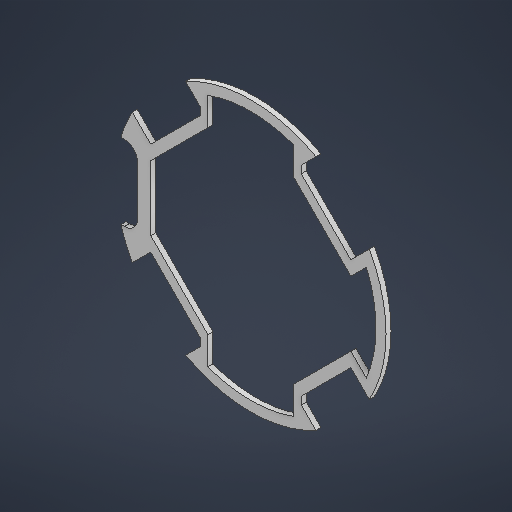
# Autodesk Inventor part: Part1
Saved by Autodesk Inventor 2026.1 (Build 301233020, 233B)
## iProperties
Created: 2026-04-01
Part Number: Part1
Material: Generic
Document SubType Name: Modeling
Designer: Bahaa
Density: 1 g/cm^3
Appearance: Default
Author: Bahaa
Autodesk Inventor part; units mm, degrees
ref_plane "YZ Plane" through (0, 0, 0) normal (1, 0, 0) x (0, 1, 0)
ref_plane "XZ Plane" through (0, 0, 0) normal (0, 1, 0) x (-1, 0, 0)
ref_plane "XY Plane" through (0, 0, 0) normal (0, 0, 1) x (1, 0, 0)
sketch "Sketch1" plane through (0, 0, 0) normal (0, 1, 0) x (-1, 0, 0)
  circle A0 centre (0, 0) radius 107.5
  line L0 (132.5, 30) -> (82.5, 30)
  line L1 (82.5, 30) -> (82.5, -30)
  line L2 (82.5, -30) -> (132.5, -30)
  line L3 (132.5, -30) -> (132.5, 30)
  line L4 (132.5, 30) -> (82.5, -30) construction
  line L5 (82.5, 30) -> (132.5, -30) construction
  line L6 (107.5, 30) -> (107.5, -30) construction
  line L7 (140.5, 38) -> (74.5, 38)
  line L8 (74.5, 38) -> (74.5, -38)
  line L9 (74.5, -38) -> (140.5, -38)
  line L10 (140.5, -38) -> (140.5, 38)
  line L11 (82.5, 0) -> (74.5, 0) construction
  line L12 (78.5, 0) -> (78.5, -18) construction
  line L13 (78.5, 0) -> (78.5, 18) construction
  line L14 (55.5079, 55.5079) -> (68.2358, 42.78) construction
  line L15 (55.5079, 55.5079) -> (42.78, 68.2358) construction
  line L16 (58.3363, 58.3363) -> (52.6795, 52.6795) construction
  line L17 (37.1231, 79.5495) -> (79.5495, 37.1231)
  line L18 (25.8094, 79.5495) -> (79.5495, 25.8094)
  line L19 (54.8008, 97.2272) -> (97.2272, 54.8008) construction
  line L20 (72.4784, 114.9049) -> (37.1231, 79.5495)
  line L21 (79.5495, 37.1231) -> (114.9049, 72.4784)
  line L22 (79.5495, 25.8094) -> (126.2186, 72.4784)
  line L23 (72.4784, 126.2186) -> (25.8094, 79.5495)
  line L24 (72.4784, 114.9049) -> (79.5495, 37.1231) construction
  line L25 (37.1231, 79.5495) -> (114.9049, 72.4784) construction
  line L26 (114.9049, 72.4784) -> (72.4784, 114.9049)
  line L27 (126.2186, 72.4784) -> (72.4784, 126.2186)
  line L28 (0, 78.5) -> (18, 78.5) construction
  line L29 (0, 78.5) -> (-18, 78.5) construction
  line L30 (0, 82.5) -> (0, 74.5) construction
  line L31 (-30, 82.5) -> (30, 82.5)
  line L32 (-38, 74.5) -> (38, 74.5)
  line L33 (-30, 107.5) -> (30, 107.5) construction
  line L34 (-30, 132.5) -> (-30, 82.5)
  line L35 (30, 82.5) -> (30, 132.5)
  line L36 (38, 74.5) -> (38, 140.5)
  line L37 (-38, 140.5) -> (-38, 74.5)
  line L38 (-30, 132.5) -> (30, 82.5) construction
  line L39 (-30, 82.5) -> (30, 132.5) construction
  line L40 (30, 132.5) -> (-30, 132.5)
  line L41 (38, 140.5) -> (-38, 140.5)
  line L42 (-55.5079, 55.5079) -> (-42.78, 68.2358) construction
  line L43 (-55.5079, 55.5079) -> (-68.2358, 42.78) construction
  line L44 (-58.3363, 58.3363) -> (-52.6795, 52.6795) construction
  line L45 (-79.5495, 37.1231) -> (-37.1231, 79.5495)
  line L46 (-79.5495, 25.8094) -> (-25.8094, 79.5495)
  line L47 (-97.2272, 54.8008) -> (-54.8008, 97.2272) construction
  line L48 (-114.9049, 72.4784) -> (-79.5495, 37.1231)
  line L49 (-37.1231, 79.5495) -> (-72.4784, 114.9049)
  line L50 (-25.8094, 79.5495) -> (-72.4784, 126.2186)
  line L51 (-126.2186, 72.4784) -> (-79.5495, 25.8094)
  line L52 (-114.9049, 72.4784) -> (-37.1231, 79.5495) construction
  line L53 (-79.5495, 37.1231) -> (-72.4784, 114.9049) construction
  line L54 (-72.4784, 114.9049) -> (-114.9049, 72.4784)
  line L55 (-72.4784, 126.2186) -> (-126.2186, 72.4784)
  line L56 (-78.5, 0) -> (-78.5, 18) construction
  line L57 (-78.5, 0) -> (-78.5, -18) construction
  line L58 (-82.5, 0) -> (-74.5, 0) construction
  line L59 (-82.5, -30) -> (-82.5, 30)
  line L60 (-74.5, -38) -> (-74.5, 38)
  line L61 (-107.5, -30) -> (-107.5, 30) construction
  line L62 (-132.5, -30) -> (-82.5, -30)
  line L63 (-82.5, 30) -> (-132.5, 30)
  line L64 (-74.5, 38) -> (-140.5, 38)
  line L65 (-140.5, -38) -> (-74.5, -38)
  line L66 (-132.5, -30) -> (-82.5, 30) construction
  line L67 (-82.5, -30) -> (-132.5, 30) construction
  line L68 (-132.5, 30) -> (-132.5, -30)
  line L69 (-140.5, 38) -> (-140.5, -38)
  line L70 (-55.5079, -55.5079) -> (-68.2358, -42.78) construction
  line L71 (-55.5079, -55.5079) -> (-42.78, -68.2358) construction
  line L72 (-58.3363, -58.3363) -> (-52.6795, -52.6795) construction
  line L73 (-37.1231, -79.5495) -> (-79.5495, -37.1231)
  line L74 (-25.8094, -79.5495) -> (-79.5495, -25.8094)
  line L75 (-54.8008, -97.2272) -> (-97.2272, -54.8008) construction
  line L76 (-72.4784, -114.9049) -> (-37.1231, -79.5495)
  line L77 (-79.5495, -37.1231) -> (-114.9049, -72.4784)
  line L78 (-79.5495, -25.8094) -> (-126.2186, -72.4784)
  line L79 (-72.4784, -126.2186) -> (-25.8094, -79.5495)
  line L80 (-72.4784, -114.9049) -> (-79.5495, -37.1231) construction
  line L81 (-37.1231, -79.5495) -> (-114.9049, -72.4784) construction
  line L82 (-114.9049, -72.4784) -> (-72.4784, -114.9049)
  line L83 (-126.2186, -72.4784) -> (-72.4784, -126.2186)
  line L84 (0, -78.5) -> (-18, -78.5) construction
  line L85 (0, -78.5) -> (18, -78.5) construction
  line L86 (0, -82.5) -> (0, -74.5) construction
  line L87 (30, -82.5) -> (-30, -82.5)
  line L88 (38, -74.5) -> (-38, -74.5)
  line L89 (30, -107.5) -> (-30, -107.5) construction
  line L90 (30, -132.5) -> (30, -82.5)
  line L91 (-30, -82.5) -> (-30, -132.5)
  line L92 (-38, -74.5) -> (-38, -140.5)
  line L93 (38, -140.5) -> (38, -74.5)
  line L94 (30, -132.5) -> (-30, -82.5) construction
  line L95 (30, -82.5) -> (-30, -132.5) construction
  line L96 (-30, -132.5) -> (30, -132.5)
  line L97 (-38, -140.5) -> (38, -140.5)
  line L98 (55.5079, -55.5079) -> (42.78, -68.2358) construction
  line L99 (55.5079, -55.5079) -> (68.2358, -42.78) construction
  line L100 (58.3363, -58.3363) -> (52.6795, -52.6795) construction
  line L101 (79.5495, -37.1231) -> (37.1231, -79.5495)
  line L102 (79.5495, -25.8094) -> (25.8094, -79.5495)
  line L103 (97.2272, -54.8008) -> (54.8008, -97.2272) construction
  line L104 (114.9049, -72.4784) -> (79.5495, -37.1231)
  line L105 (37.1231, -79.5495) -> (72.4784, -114.9049)
  line L106 (25.8094, -79.5495) -> (72.4784, -126.2186)
  line L107 (126.2186, -72.4784) -> (79.5495, -25.8094)
  line L108 (114.9049, -72.4784) -> (37.1231, -79.5495) construction
  line L109 (79.5495, -37.1231) -> (72.4784, -114.9049) construction
  line L110 (72.4784, -114.9049) -> (114.9049, -72.4784)
  line L111 (72.4784, -126.2186) -> (126.2186, -72.4784)
  circle A1 centre (0, 0) radius 99.5
  line L112 (37.1231, 79.5495) -> (34.1231, 79.5495) construction
  line L113 (34.1231, 79.5495) -> (34.1231, 71.2358)
  line L114 (34.1231, 79.5495) -> (34.1231, 93.4658)
  line L115 (37.1231, 79.5495) -> (40.1231, 79.5495) construction
  line L116 (40.1231, 79.5495) -> (40.1231, 82.5495)
  line L117 (40.1231, 79.5495) -> (40.1231, 76.5495)
  line L118 (-34.1231, 79.5495) -> (-34.1231, 71.2358)
  line L119 (-34.1231, 79.5495) -> (-34.1231, 93.4658)
  line L120 (-40.1231, 79.5495) -> (-40.1231, 82.5495)
  line L121 (-40.1231, 79.5495) -> (-40.1231, 76.5495)
  line L122 (34.1231, -79.5495) -> (34.1231, -71.2358)
  line L123 (34.1231, -79.5495) -> (34.1231, -93.4658)
  line L124 (40.1231, -79.5495) -> (40.1231, -82.5495)
  line L125 (40.1231, -79.5495) -> (40.1231, -76.5495)
  line L126 (-34.1231, -79.5495) -> (-34.1231, -93.4658)
  line L127 (-34.1231, -79.5495) -> (-34.1231, -71.2358)
  line L128 (-40.1231, -79.5495) -> (-40.1231, -82.5495)
  line L129 (-40.1231, -79.5495) -> (-40.1231, -76.5495)
  point P0 (107.5, 0)
  point P1 (76.014, 76.014)
  point P2 (0, 107.5)
  point P3 (-76.014, 76.014)
  point P4 (-107.5, 0)
  point P5 (-76.014, -76.014)
  point P6 (0, -107.5)
  point P7 (76.014, -76.014)
  point P8 (91.8941, 38.154)
  point P9 (91.8941, -38.154)
  point P10 (38.154, -91.8941)
  point P11 (-38.154, -91.8941)
  point P12 (-91.8941, -38.154)
  point P13 (-91.8941, 38.154)
  point P14 (-38.154, 91.8941)
  point P15 (38.154, 91.8941)
  point P16 (94.2072, 51.7808)
  point P17 (51.7808, 94.2072)
  point P18 (-51.7808, 94.2072)
  point P19 (-94.2072, 51.7808)
  point P20 (-94.2072, -51.7808)
  point P21 (-51.7808, -94.2072)
  point P22 (51.7808, -94.2072)
  point P23 (94.2072, -51.7808)
  point P24 (88.2962, -45.8698)
  point P25 (45.8698, -88.2962)
  point P26 (45.8698, 88.2962)
  point P27 (88.2962, 45.8698)
  point P28 (44.2364, -97.9765)
  point P29 (97.9765, -44.2364)
  point P30 (97.9765, 44.2364)
  point P31 (44.2364, 97.9765)
  point P32 (-45.8698, -88.2962)
  point P33 (-88.2962, -45.8698)
  point P34 (-88.2962, 45.8698)
  point P35 (-45.8698, 88.2962)
  point P36 (-97.9765, -44.2364)
  point P37 (-44.2364, -97.9765)
  point P38 (-44.2364, 97.9765)
  point P39 (-97.9765, 44.2364)
  dimension "d0" = 215
  dimension "d10" = 8
  dimension "d2" = 60
  dimension "d3" = 50
  dimension "d4" = 8
  dimension "d5" = 18
  dimension "d8" = 360
  dimension "d39" = 3
  dimension "d40" = 3
  constraints: 260 end point, 20 symmetric about line, 11 coincident, 7 midpoint, 6 vertical, 4 parallel, 3 horizontal, 3 point on line, 2 perpendicular, 266 other
  measures "d2" distance of L1.end L0.end
  measures "d3" diameter of L1 L6
  measures "d4" distance between parallel lines of L3 L10
  measures "d5" distance of L12.start L12.end
  measures "d39" distance of L17.start L112.end
  measures "d40" distance of L17.start L115.end
extrude "Extrusion1" add sketch "Sketch1" against normal blind 4 contours L22 A1 L21 A0 | L22 L1 L0 | L0 L1 L22 L18 L8 L7 L17 L21 | A0 L104 A1 L107 | L107 L9 L104 L101 L8 L102 L1 L2 | L2 L1 L107 | L22 L7 L21 A1 | A1 L104 L9 L107 | L20 A1 L23 A0 | A0 L106 A1 L105 | L23 A1 L36 A0 | L20 L36 L23 A1 | L7 L8 L18 L113 L32 L36 L17 | A0 L93 A1 L106 | A1 L106 L93 L105 | L101 L93 L88 L122 L102 L8 L9 | L36 A1 L35 A0 | L23 L36 A1 | L116 L117 L17 L36 L20 | A0 L90 A1 L93 | A1 L93 L106 | L105 L93 L101 L125 L124 | L35 A1 L34 A0 | L36 L23 L114 A1 | L36 L20 L17 L32 L113 L114 L23 | L36 L17 L20 | A0 L91 A1 L90 | A1 L123 L106 L93 | L106 L123 L122 L88 L93 L101 L105 | L105 L101 L93 | L34 A1 L37 A0 | A0 L92 A1 L91 | L37 A1 L50 A0 | L118 L46 L60 L64 L45 L37 L32 | L32 L37 L45 L49 L50 L119 L118 | A0 L79 A1 L92 | L127 L88 L92 L73 L65 L60 L74 | L127 L126 L79 L92 L76 L73 L88 | L50 A1 L49 A0 | A1 L119 L50 L37 | L37 L50 A1 | L46 L51 L59 L63 L64 L48 L45 L60 | A0 L76 A1 L79 | A1 L79 L92 | L92 L79 L126 A1 | L60 L65 L73 L77 L78 L62 L59 L74 | L50 L37 L49 A1 | L45 L121 L120 L49 L37 | L37 L49 L45 | A1 L76 L92 L79 | L92 L76 L128 L129 L73 | L73 L76 L92 | L48 A1 L51 A0 | L51 L63 L59 | A0 L78 A1 L77 | L59 L62 L78 | L51 A1 L64 A0 | L48 L64 L51 A1 | A0 L65 A1 L78 | A1 L78 L65 L77 | L64 A1 L63 A0 | A1 L62 A0 L63 | A0 L62 A1 L65
sketch "Sketch2" plane through (0, 0, 0) normal (0, 1, 0) x (1, 0, 0)
  arc A0 (34.1231, 93.4658) -> (-34.1231, 93.4658) centre (0, 0) ccw projected
  arc A1 (-94.2072, 51.7808) -> (-94.2072, -51.7808) centre (0, 0) ccw projected
  arc A2 (34.1231, 93.4658) -> (-34.1231, 93.4658) centre (0, 0) ccw projected
  line L0 (-90, 0) -> (-90, 19.5)
  line L1 (-102.5, -32.4037) -> (-102.5, 32.4037) construction
  line L2 (-100.5, 30) -> (-102.5, 30)
  line L3 (-90, 0) -> (-107.5, 0) construction
  line L4 (-90, 0) -> (-90, -19.5)
  line L5 (-100.5, -30) -> (-102.5, -30)
  line L6 (-102.5, -30) -> (-103.2291, -30)
  line L7 (-102.5, 30) -> (-103.2291, 30)
  line L8 (-79.5495, -25.8094) -> (-79.5495, 25.8094)
  line L9 (-97.9765, 44.2364) -> (-79.5495, 25.8094) projected
  line L10 (-79.5495, -25.8094) -> (-97.9765, -44.2364) projected
  arc A3 (-90, 19.5) -> (-100.5, 30) centre (-100.5, 19.5) ccw
  arc A4 (-100.5, -30) -> (-90, -19.5) centre (-100.5, -19.5) ccw
  point P0 (-102.5, 0)
  point P1 (99.5, 0)
  point P2 (99.5, 0)
  point P3 (-103.2291, -30)
  point P4 (-103.2291, 30)
  point P5 (-95.2953, 28.6193)
  point P6 (-95.2953, -28.6193)
  dimension "d21" = 5
  dimension "d22" = 2
  dimension "d27" = 60
  dimension "d35" = 12.5
  dimension "d37" = 10.5
  constraints: 18 end point, 6 point on circle, 4 symmetric about line, 3 horizontal, 2 centre point, 2 vertical, 1 midpoint, 1 perpendicular, 1 point on line, 1 tangent, 7 other
  measures "d21" distance of L3.end point (-102.5, 0)
  measures "d22" distance of L2.start L2.end
  measures "d27" diameter of L2.start L3
  measures "d35" distance between parallel lines of L1 L0
  measures "d37" radius of A3
extrude "Extrusion2" add sketch "Sketch2" against normal blind 4 contours L9 L8 L10 A1 L6 L5 A4 L4 L0 A3 L2 L7
extrude "Extrusion3" [suppressed]
equation "\"d37\" = d35 - d22"
body "Solid1"
